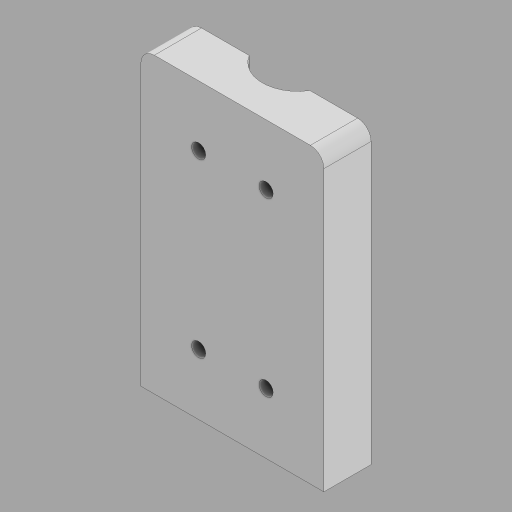
# Autodesk Inventor part: end_arm_수정
Saved by Autodesk Inventor 2023.1 (Build 271208000, 208)
## iProperties
Created: 2022-10-28
Part Number: end_arm_수정
Material: 일반
Document SubType Name: Modeling
Designer: 박동준
Density: 1 g/cm^3
Appearance: 기본값
품번: 22
Author: 박동준
Autodesk Inventor part; units mm, degrees
ref_plane "YZ Plane" through (0, 0, 0) normal (1, 0, 0) x (0, 1, 0)
ref_plane "XZ Plane" through (0, 0, 0) normal (0, 1, 0) x (-1, 0, 0)
ref_plane "XY Plane" through (0, 0, 0) normal (0, 0, 1) x (1, 0, 0)
sketch "스케치1" plane through (0, 0, 0) normal (1, 0, 0) x (0, 1, 0)
  line L0 (21.75, 7) -> (-21.75, 7)
  line L1 (-21.75, 7) -> (-21.75, 0)
  line L2 (-21.75, 0) -> (-3.25, 0)
  line L3 (-3.25, 0) -> (-3.25, 0)
  line L4 (-3.25, 0) -> (21.75, 0)
  line L5 (21.75, 0) -> (21.75, 7)
  point P0 (0, 0)
  point P1 (0, 7)
  dimension "d0" = 43.5
  dimension "d1" = 25
  dimension "d2" = 7
  dimension "d3" = 7
  constraints: 12 end point, 5 perpendicular, 1 horizontal, 1 horizontal alignment, 1 midpoint, 1 vertical alignment
  measures "d0" distance of L0.start L0.end
  measures "d1" distance of L3.end L4.end
  measures "d2" distance of L4.end L0.start
  measures "d3" distance of L0.end L1.end
extrude "돌출1" add sketch "스케치1" along normal mid plane 27.14
sketch "스케치2" plane through (13.57, 21.75, 0) normal (0, 0, -1) x (-1, 0, 0)
  circle A0 centre (8.57, -9) radius 1.05
  circle A1 centre (18.57, -9) radius 1.05
  circle A2 centre (8.57, -34.5) radius 1.05
  circle A3 centre (18.57, -34.5) radius 1.05
  line L0 (8.57, -9) -> (18.57, -9) construction
  line L1 (8.57, -34.5) -> (18.57, -34.5) construction
  line L2 (27.14, -43.5) -> (0, -43.5) projected
  point P0 (13.57, -21.75)
  point P1 (13.57, -34.5)
  point P2 (13.57, -9)
  dimension "d41" = 2.1
  dimension "d42" = 2.1
  dimension "d43" = 2.1
  dimension "d44" = 2.1
  dimension "d45" = 25.5
  dimension "d46" = 9
  dimension "d47" = 10
  dimension "d48" = 10
  constraints: 4 centre point, 4 end point, 2 horizontal, 2 midpoint, 2 vertical alignment
  measures "d41" diameter of A0
  measures "d42" diameter of A1
  measures "d43" diameter of A2
  measures "d44" diameter of A3
  measures "d45" distance between parallel lines of L1 L0
  measures "d46" distance between parallel lines of L2 L1
  measures "d47" distance of L0.start L0.end
  measures "d48" distance of L1.start L1.end
extrude "돌출2" cut sketch "스케치2" against normal through all
sketch "스케치3" plane through (13.57, 21.75, 0) normal (0, 0, -1) x (-1, 0, 0)
  circle A0 centre (18.57, -34.5) radius 1.05 projected
  circle A1 centre (18.57, -9) radius 1.05 projected
  circle A2 centre (8.57, -34.5) radius 1.05 projected
  circle A3 centre (8.57, -9) radius 1.05 projected
  line L0 (27.14, 0) -> (0, 0) projected
  line L1 (0, -43.5) -> (0, 0) projected
  line L2 (27.14, -43.5) -> (0, -43.5) projected
  line L3 (27.14, 0) -> (27.14, -43.5) projected
  circle A4 centre (8.57, -9) radius 1.05 projected
  circle A5 centre (8.57, -9) radius 2.25
  circle A6 centre (18.57, -9) radius 2.25
  circle A7 centre (8.57, -34.5) radius 1.05 projected
  circle A8 centre (8.57, -34.5) radius 2.25
  circle A9 centre (18.57, -34.5) radius 2.25
  point P0 (13.57, -21.75)
  dimension "d51" = 4.5
  dimension "d52" = 4.5
  dimension "d53" = 4.5
  dimension "d54" = 4.5
  constraints: 4 centre point, 4 coincident
  measures "d51" diameter of A5
  measures "d52" diameter of A6
  measures "d53" diameter of A8
  measures "d54" diameter of A9
extrude "돌출3" cut sketch "스케치3" against normal blind 4 contours A5 | A6 | A8 | A9
sketch "스케치4" plane through (-13.57, -21.75, 0) normal (0, -1, 0) x (1, 0, 0)
  circle A0 centre (13.57, -2.7) radius 5.25
  line L0 (0, 0) -> (27.14, 0) projected
  line L1 (0, 0) -> (27.14, 0) projected
  point P0 (13.57, 0)
  point P1 (13.57, 0)
  point P2 (13.57, 0)
  dimension "d67" = 10.5
  dimension "d68" = 2.7
  constraints: 2 midpoint, 2 vertical alignment, 1 centre point
  measures "d67" diameter of A0
  measures "d68" distance from line of L0 A0.centre
extrude "돌출4" cut sketch "스케치4" against normal through all
sketch "스케치5" plane through (13.57, -21.75, 0) normal (0, 0, -1) x (-1, 0, 0)
  line L0 (9.0675, 0) -> (9.0675, 6.8057) projected
  arc A0 (9.0675, 11.1943) -> (9.0675, 6.8057) centre (8.57, 9) ccw projected
  line L1 (9.0675, 11.1943) -> (9.0675, 32.3057) projected
  arc A1 (9.0675, 36.6943) -> (9.0675, 32.3057) centre (8.57, 34.5) ccw projected
  line L2 (9.0675, 36.6943) -> (9.0675, 43.5) projected
  line L3 (9.0675, 43.5) -> (0, 43.5) projected
  line L4 (0, 0) -> (0, 43.5) projected
  line L5 (9.0675, 0) -> (0, 0) projected
  circle A2 centre (3.4, 26.75) radius 1.4
  circle A3 centre (3.4, 16.75) radius 1.4
  line L6 (9.0675, 0) -> (0, 0) projected
  point P0 (13.57, 21.75)
  point P1 (4.5338, 0)
  point P2 (4.5338, 0)
  dimension "d71" = 2.8
  dimension "d72" = 2.8
  dimension "d78" = 3.4
  dimension "d79" = 26.75
  dimension "d80" = 16.75
  constraints: 2 centre point, 2 midpoint, 1 vertical alignment
  measures "d71" diameter of A2
  measures "d72" diameter of A3
  measures "d78" distance from line of L4 A3.centre
  measures "d79" distance from line of A2.centre L5
  measures "d80" distance from line of L5 A3.centre
extrude "돌출5" cut sketch "스케치5" against normal blind 5 contours A2 | A3
mirror "미러1" about plane through (0, 0, 0) normal (1, 0, 0) of "돌출5"
fillet "모깎기2" radius 2 2 edges at (13.57, 21.75, 3.5) (-13.57, 21.75, 3.5)
ref_plane "작업 평면1" through (0, 0, 0) normal (1, 0, 0) x (0, 1, 0)
